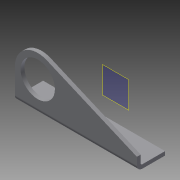
# Autodesk Inventor part: Flange Bearing Mount Tower Mirror
Saved by Autodesk Inventor 2013 (Build 170138000, 138)
## iProperties
Created: 2013-01-21
Part Number: Flange Bearing Mount Tower Mirror
Material: Generic
Document SubType Name: Sheet Metal
Designer: actoennies
Density: 1 g/cm^3
Sheet Metal Rule: Default
Mass: 13.7818 g
Surface Area: 100.387 cm^2
Volume: 13.7818 cm^3
Flat Pattern Width: 6.32443 cm
Flat Pattern Length: 10.16 cm
Flat Pattern Area: 64.2562 cm^2
Sheet Metal Width: 2.490 in
Sheet Metal Length: 4.000 in
Sheet Metal Area: 9.960 in^2
Author: actoennies
Autodesk Inventor part; units mm, degrees
ref_plane "YZ Plane" through (0, 0, 0) normal (1, 0, 0) x (0, 1, 0)
ref_plane "XZ Plane" through (0, 0, 0) normal (0, 1, 0) x (-1, 0, 0)
ref_plane "XY Plane" through (0, 0, 0) normal (0, 0, 1) x (1, 0, 0)
sketch "Sketch1" plane through (0, 0, 0) normal (0, 1, 0) x (-1, 0, 0)
  line L0 (0, 0) -> (-76.2, 0)
  line L1 (0, 0) -> (-12.7, 0)
  circle A0 centre (-38.1, 6.35) radius 3.3782
  circle A1 centre (-63.5, 6.35) radius 3.3782
  line L2 (0, 0) -> (0, 19.05)
  line L3 (0, 19.05) -> (-101.6, 19.05)
  line L4 (-101.6, 19.05) -> (-101.6, 0)
  line L5 (-101.6, 0) -> (-76.2, 0)
  dimension "d2" = 6.7564
  dimension "d3" = 6.7564
  dimension "d26" = 19.05
  dimension "d27" = 101.6
  measures "d2" diameter of A0
  measures "d3" diameter of A1
  measures "d26" distance of L0.start L2.end
  measures "d27" distance of L2.end L3.end
extrude "Plate1" add sketch "Sketch1" along normal blind 3.175
ref_plane "Work Plane1" through (76.2, 44.45, 15.875) normal (0, 0, -1) x (-1, 0, 0)
sketch "Sketch4" plane through (101.6, 4.445, 20.32) normal (0, 0, 1) x (1, 0, 0)
  line L0 (-101.6, 0) -> (0, 0)
  line L1 (0, 0) -> (0, 40.005)
  line L2 (0, 40.005) -> (-101.6, 40.005)
  line L3 (-101.6, 40.005) -> (-101.6, 0)
  constraints: 6 end point, 1 horizontal, 1 perpendicular, 1 vertical
edge flange "Flange2" height 44.45 angle 90 thickness 3.175 bend radius 1.27 thickness toward (0, 0, 1) relief straight relief width 3.175 relief depth 1.5875 edges at (50.8, 3.175, 19.05) wall of the first edge with corners at (0, 4.445, 20.32) (101.6, 4.445, 20.32) (101.6, 44.45, 20.32) (0, 44.45, 20.32)
bend "Bend2"
corner "Corner2"
sketch "Sketch5" plane through (101.6, 44.45, 20.32) normal (0, 0, -1) x (-1, 0, 0)
  circle A0 centre (82.55, -19.05) radius 14.2875 projected
  line L0 (0, -40.005) -> (101.6, -40.005) projected
  line L1 (101.6, 0) -> (101.6, -40.005) projected
  line L2 (101.6, 0) -> (0, 0) projected
  line L3 (0, 0) -> (0, -40.005) projected
  line L4 (0, -40.005) -> (0, -33.655)
  arc A1 (101.6, -19.05) -> (75.0553, -1.5363) centre (82.55, -19.05) ccw
  line L5 (0, -33.655) -> (75.0553, -1.5363)
  point P0 (101.6, -44.45)
  dimension "d42" = 6.35
  constraints: 4 end point, 2 point on circle, 2 point on line, 2 tangent, 1 centre point, 1 coincident
  measures "d42" distance of L0.start L4.end
extrude "Cut3" cut sketch "Sketch5" against normal blind 3.175 contours L3 L2 A1 L5 | A1 L2 L1
sketch "Sketch6" plane through (0, 3.175, 0) normal (0, 1, 0) x (1, 0, 0)
  circle A0 centre (63.5, -6.35) radius 3.3782
  circle A1 centre (38.1, -6.35) radius 3.3782
  circle A2 centre (38.1, -6.35) radius 3.3782
  circle A3 centre (63.5, -6.35) radius 3.3782
sheet face with bend "Face2" sketch "Sketch6" thickness 3.175 toward (0, -1, 0) bend radius 3.175 relief straight relief width 3.175 relief depth 1.5875
bend "Bend3"
sketch "Sketch7" plane through (0, 3.175, 0) normal (0, 1, 0) x (1, 0, 0)
  circle A0 centre (57.15, -12.7) radius 3.3782 projected
  circle A1 centre (79.375, -12.7) radius 3.3782 projected
extrude "Cut4" cut sketch "Sketch7" against normal blind 3.175
sketch "Sketch8" plane through (101.6, 4.445, 20.32) normal (0, 0, -1) x (-1, 0, 0)
  arc A0 (101.6, 20.955) -> (75.0553, 38.4687) centre (82.55, 20.955) ccw projected
  circle A1 centre (82.55, 20.955) radius 14.2875
  point P0 (101.6, -4.445)
  dimension "d52" = 28.575
  constraints: 1 centre point, 1 coincident
  measures "d52" diameter of A1
extrude "Cut5" cut sketch "Sketch8" against normal blind 3.175
equation "\"d43\" = Thickness"
equation "\"d50\" = Thickness"
equation "\"d53\" = Thickness"
equation "\"d28\" = BendReliefWidth"
equation "\"d29\" = BendReliefDepth"
equation "\"d30\" = MinimumRemnant"
equation "\"d31\" = BendRadius"
equation "\"d35\" = CornerReliefSize"
equation "\"d36\" = GapSize"
equation "\"d37\" = JacobiRadiusSize"
equation "\"d45\" = BendRadius"
equation "\"d46\" = BendReliefWidth"
equation "\"d48\" = MinimumRemnant"
equation "\"d47\" = BendReliefDepth"
equation "\"d49\" = BendRadius"
equation "\"BendRadius\" = Thickness"
equation "\"BendReliefWidth\" = Thickness"
equation "\"BendReliefDepth\" = 0.5 * Thickness"
equation "\"CornerReliefSize\" = 4 * Thickness"
equation "\"MinimumRemnant\" = 2 * Thickness"
equation "\"TransitionRadius\" = BendRadius"
equation "\"JacobiRadiusSize\" = BendRadius"
equation "\"GapSize\" = Thickness"
equation "\"d9\" = BendRadius"
equation "\"Thickness\" = 3.175"
body "Solid1"
